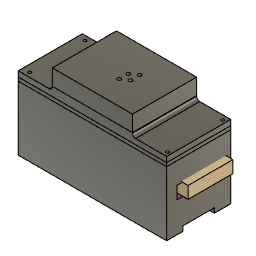
Enphase Relay Controller Unit v24 (Autodesk Fusion 360 design; units mm, degrees)
Autodesk Fusion 360 part; units mm, degrees
sketch "Device 1" plane through (0, 0, 0) normal (0, 0, 1) x (1, 0, 0)
  line L0 (0, 0) -> (58, 0)
  line L1 (58, 0) -> (58, 29)
  line L2 (58, 29) -> (0, 29)
  line L3 (0, 29) -> (0, 0)
  dimension "d1" = 58
  dimension "d2" = 29
  constraint horizontal L0
  constraint vertical L1
  constraint horizontal L2
  constraint vertical L3
  constraint coincident L0.start L3.end
  measures "d1" distance of L0.start L0.end
  measures "d2" distance of L0.start L2.end
extrude "Extrude1" add sketch "Device 1" along normal blind 1.5 makes body 1
sketch "Device 2" plane through (0, 0, 1.5) normal (0, 0, 1) x (-1, 0, 0)
  line L0 (0, -29) -> (0, 0)
  line L1 (0, 0) -> (-58, 0)
  line L2 (-58, 0) -> (-58, -29)
  line L3 (-58, -29) -> (0, -29)
  line L4 (0, -29) -> (-5, -29) construction
  line L5 (-5, -29) -> (-5, -28) construction
  line L6 (-5, -28) -> (-53, -28)
  line L7 (-53, -28) -> (-53, -25.7)
  line L8 (-53, -25.7) -> (-5, -25.7)
  line L9 (-5, -25.7) -> (-5, -28)
  line L10 (0, 0) -> (-5, 0) construction
  line L11 (-5, 0) -> (-5, -1) construction
  line L12 (-5, -1) -> (-53, -1)
  line L13 (-53, -1) -> (-53, -3.3)
  line L14 (-53, -3.3) -> (-5, -3.3)
  line L15 (-5, -3.3) -> (-5, -1)
  line L16 (-58, -29) -> (-58, -24) construction
  line L17 (-58, 0) -> (-58, -13) construction
  line L18 (-58, -24) -> (-55, -24) construction
  line L19 (-58, -13) -> (-59.5, -13) construction
  line L20 (-55, -24) -> (-59.5, -24)
  line L21 (-59.5, -24) -> (-59.5, -13)
  line L22 (-59.5, -13) -> (-55, -13)
  line L23 (-55, -13) -> (-55, -24)
  dimension "d5" = 5
  dimension "d6" = 1
  dimension "d9" = 48
  dimension "d10" = 2.3
  dimension "d11" = 5
  dimension "d12" = 1
  dimension "d13" = 48
  dimension "d14" = 2.3
  dimension "d99" = 5
  dimension "d100" = 13
  dimension "d101" = 3
  dimension "d102" = 1.5
  constraint coincident L0.start L3.end
  constraint perpendicular L0 L4
  constraint perpendicular L4 L5
  constraint horizontal L6
  constraint vertical L7
  constraint horizontal L8
  constraint vertical L9
  constraint coincident L0.end L1.start
  constraint coincident L1 L10.end
  constraint perpendicular L10 L11
  constraint horizontal L12
  constraint vertical L13
  constraint horizontal L14
  constraint vertical L15
  constraint coincident L2.end L3.start
  constraint perpendicular L3 L16
  constraint coincident L1.end L2.start
  constraint perpendicular L1 L17
  constraint perpendicular L2 L18
  constraint perpendicular L17 L19
  constraint horizontal L20
  constraint vertical L21
  constraint horizontal L22
  constraint vertical L23
  measures "d5" distance of L0.start L4.end
  measures "d6" distance of L4.end L5.end
  measures "d9" distance of L5.end L6.end
  measures "d10" distance of L5.end L8.end
  measures "d11" distance of L0.end L10.end
  measures "d12" distance of L10.end L11.end
  measures "d13" distance of L11.end L12.end
  measures "d14" distance of L11.end L14.end
  measures "d99" distance of L2.end L16.end
  measures "d100" distance of L1.end L17.end
  measures "d101" distance of L16.end L18.end
  measures "d102" distance of L17.end L19.end
extrude "Extrude2" add sketch "Device 2" along normal blind 11.12 contours L6 L7 L8 L9 | L12 L13 L14 L15 bodies 1
sketch "Device 3" plane through (0, 0, 12.62) normal (0, 0, 1) x (-1, 0, 0)
  line L0 (-5, -3.3) -> (-5, -1)
  line L1 (-5, -1) -> (-53, -1)
  line L2 (-53, -1) -> (-53, -3.3)
  line L3 (-53, -3.3) -> (-5, -3.3)
  line L4 (-5, -1) -> (-0.8, -1) construction
  line L5 (-0.8, -1) -> (-0.8, 0.45) construction
  line L6 (-0.8, 0.45) -> (-57.6, 0.45)
  line L7 (-57.6, 0.45) -> (-57.6, -31.05)
  line L8 (-57.6, -31.05) -> (-0.8, -31.05)
  line L9 (-0.8, -31.05) -> (-0.8, 0.45)
  line L10 (-57.6, 0.45) -> (-57.6, -4.72) construction
  line L11 (-57.6, -4.72) -> (-67.2, -4.72)
  line L12 (-67.2, -4.72) -> (-67.2, -29.82)
  line L13 (-67.2, -29.82) -> (-57.6, -29.82)
  line L14 (-57.6, -29.82) -> (-57.6, -4.72)
  dimension "d17" = 4.2
  dimension "d18" = 1.45
  dimension "d19" = 56.8
  dimension "d20" = 31.5
  dimension "d21" = 5.17
  dimension "d22" = 9.6
  dimension "d23" = 25.1
  constraint coincident L0.end L1.start
  constraint perpendicular L0 L4
  constraint perpendicular L4 L5
  constraint horizontal L6
  constraint vertical L7
  constraint horizontal L8
  constraint vertical L9
  constraint perpendicular L6 L10
  constraint horizontal L11
  constraint vertical L12
  constraint horizontal L13
  constraint vertical L14
  measures "d17" distance of L0.end L4.end
  measures "d18" distance of L4.end L5.end
  measures "d19" distance of L5.end L6.end
  measures "d20" distance of L5.end L8.end
  measures "d21" distance of L6.end L10.end
  measures "d22" distance of L10.end L11.end
  measures "d23" distance of L10.end L13.end
extrude "Extrude3" add sketch "Device 3" along normal blind 1.6 contours L0 L1 L2 L3 | L6 L7 L8 L9 L14 bodies 1
extrude "Extrude4" add sketch "Device 3" along normal blind 5.77 contours L7 L11 L12 L13 L14 bodies 1
sketch "Device 4" plane through (0, 0, 14.22) normal (0, 0, 1) x (-1, 0, 0)
  line L0 (-57.6, -31.05) -> (-0.8, -31.05)
  line L1 (-0.8, -31.05) -> (-0.8, 0.45)
  line L2 (-0.8, 0.45) -> (-57.6, 0.45)
  line L3 (-57.6, 0.45) -> (-57.6, -4.72)
  line L4 (-57.6, -4.72) -> (-57.6, -29.82)
  line L5 (-57.6, -29.82) -> (-57.6, -31.05)
  line L6 (-57.6, -31.05) -> (-53.8, -31.05) construction
  line L7 (-53.8, -31.05) -> (-53.8, -29.25) construction
  line L8 (-53.8, -29.25) -> (-23.9, -29.25)
  line L9 (-23.9, -29.25) -> (-23.9, -8.75)
  line L10 (-23.9, -8.75) -> (-53.8, -8.75)
  line L11 (-53.8, -8.75) -> (-53.8, -29.25)
  line L12 (-53.8, -29.25) -> (-16, -29.25) construction
  line L13 (-16, -29.25) -> (-21.5, -29.25)
  line L14 (-21.5, -29.25) -> (-21.5, -17.75)
  line L15 (-21.5, -17.75) -> (-16, -17.75)
  line L16 (-16, -17.75) -> (-16, -29.25)
  line L17 (-21.5, -29.25) -> (-8.15, -29.25) construction
  line L18 (-8.15, -29.25) -> (-14, -29.25)
  line L19 (-14, -29.25) -> (-14, -14.45)
  line L20 (-14, -14.45) -> (-8.15, -14.45)
  line L21 (-8.15, -14.45) -> (-8.15, -29.25)
  dimension "d28" = 3.8
  dimension "d29" = 1.8
  dimension "d30" = 29.9
  dimension "d31" = 20.5
  dimension "d32" = 37.8
  dimension "d33" = 5.5
  dimension "d34" = 11.5
  dimension "d35" = 13.35
  dimension "d36" = 5.85
  dimension "d37" = 14.8
  constraint coincident L0.start L5.end
  constraint perpendicular L5 L6
  constraint perpendicular L6 L7
  constraint horizontal L8
  constraint vertical L9
  constraint horizontal L10
  constraint vertical L11
  constraint perpendicular L7 L12
  constraint horizontal L13
  constraint vertical L14
  constraint horizontal L15
  constraint vertical L16
  constraint perpendicular L14 L17
  constraint horizontal L18
  constraint vertical L19
  constraint horizontal L20
  constraint vertical L21
  measures "d28" distance of L0.start L6.end
  measures "d29" distance of L6.end L7.end
  measures "d30" distance of L7.end L8.end
  measures "d31" distance of L7.end L10.end
  measures "d32" distance of L7.end L12.end
  measures "d33" distance of L12.end L13.end
  measures "d34" distance of L12.end L15.end
  measures "d35" distance of L13.end L17.end
  measures "d36" distance of L17.end L18.end
  measures "d37" distance of L17.end L20.end
extrude "Extrude5" add sketch "Device 4" along normal blind 14.6 contours L8 L9 L10 L11 bodies 1
extrude "Extrude6" add sketch "Device 4" along normal blind 10.2 contours L13 L14 L15 L16 bodies 1
extrude "Extrude7" add sketch "Device 4" along normal blind 10.2 contours L18 L19 L20 L21 bodies 1
sketch "Enclosure Base 1" plane through (0, 0, 0) normal (0, 0, 1) x (1, 0, 0)
  line L0 (0, 0) -> (83.3, 0)
  line L1 (83.3, 0) -> (83.3, 35)
  line L2 (83.3, 35) -> (0, 35)
  line L3 (0, 35) -> (0, 0)
  line L4 (83.3, 17.5) -> (83.3, 26.35) construction
  line L5 (83.3, 17.5) -> (83.3, 8.65) construction
  line L6 (83.3, 26.35) -> (0, 26.35)
  line L7 (0, 26.35) -> (0, 8.65)
  line L8 (0, 8.65) -> (83.3, 8.65)
  line L9 (83.3, 8.65) -> (83.3, 26.35)
  dimension "d44" = 83.3
  dimension "d45" = 35
  dimension "d46" = 8.85
  dimension "d47" = 8.85
  constraint horizontal L0
  constraint vertical L1
  constraint horizontal L2
  constraint vertical L3
  constraint coincident L0.start L3.end
  constraint midpoint L1 L4.start
  constraint perpendicular L2 L4
  constraint parallel L1 L5
  constraint horizontal L6
  constraint vertical L7
  constraint horizontal L8
  constraint vertical L9
  constraint coincident L3 L7.end
  measures "d44" distance of L0.start L0.end
  measures "d45" distance of L0.start L2.end
  measures "d46" distance of L4.start L4.end
  measures "d47" distance of L4.start L5.end
extrude "Extrude8" add sketch "Enclosure Base 1" along normal blind 5 separate body makes body 2
extrude "Extrude9" cut sketch "Enclosure Base 1" along normal blind 2.68 contours L1 L3 L6 L7 L8 L9 bodies 2
move_body "Move1" bodies 1 to x (1, 0, 0) y (0, 1, 0) z (0, 0, 1) at (25.3, 0, 5)
extrude "Extrude10" add 1 faces at (27.7667, 0, 1.6667) along direction (0, -1, 0) blind 0.5 on bodies 2 bodies 2
extrude "Extrude11" add 1 faces at (55.5333, 35, 1.6667) along direction (0, 1, 0) blind 0.5 on bodies 2 bodies 2
move_body "Move2" bodies 1 to x (1, 0, 0) y (0, 1, 0) z (0, 0, 1) at (-5.25, 2.12, 0)
sketch "Enclosure Base 2" plane through (0, 0, 5) normal (0, 0, 1) x (-1, 0, 0)
  line L0 (-83.3, 0.5) -> (-83.3, -35.5)
  line L1 (-83.3, -35.5) -> (0, -35.5)
  line L2 (0, -35.5) -> (0, 0.5)
  line L3 (0, 0.5) -> (-83.3, 0.5)
  line L4 (-20.05, -31.12) -> (-20.05, -35.5) construction
  line L5 (-20.05, -2.12) -> (-20.05, 0.5) construction
  line L6 (-78.05, -2.12) -> (-78.05, 0.5) construction
  line L7 (-78.05, -2.12) -> (-78.3, -2.123) construction
  line L8 (-20.05, -31.12) -> (-20.05, -31.37) construction
  line L9 (-20.05, -31.37) -> (-19.8, -31.37) construction
  line L10 (-20.05, -2.12) -> (-20.05, -1.87) construction
  line L11 (-20.05, -1.87) -> (-19.8, -1.87) construction
  line L12 (-78.05, 0.5) -> (-78.05, -35.5) construction
  line L13 (0, -4.123) -> (-5, -4.123) construction
  line L14 (-19.8, -2.123) -> (-19.8, -2.823) construction
  line L15 (-19.8, -31.37) -> (-19.8, -32.07) construction
  line L16 (-78.3, -2.123) -> (-78.3, -2.823) construction
  line L17 (-5, -4.123) -> (-5, -4.823) construction
  line L18 (-19.8, -32.07) -> (-78.3, -32.07)
  line L19 (-78.3, -32.07) -> (-78.3, -2.823)
  line L20 (-78.3, -2.823) -> (-19.8, -2.823)
  line L21 (-19.8, -32.07) -> (-19.8, -2.823)
  line L22 (-19.8, -2.823) -> (-19.8, -4.823) construction
  line L23 (-19.8, -32.07) -> (-19.8, -30.07) construction
  line L24 (-19.8, -30.07) -> (-5, -30.07)
  line L25 (-5, -30.07) -> (-5, -4.823)
  line L26 (-5, -4.823) -> (-19.8, -4.823)
  line L27 (-19.8, -4.823) -> (-19.8, -30.07)
  line L28 (-19.8, -4.823) -> (-9.8, -4.823) construction
  line L29 (-19.8, -30.07) -> (-9.8, -30.07) construction
  line L30 (-9.8, -30.07) -> (-19.8, -30.07)
  line L31 (-19.8, -30.07) -> (-19.8, -32.07)
  line L32 (-19.8, -32.07) -> (-9.8, -32.07)
  line L33 (-9.8, -32.07) -> (-9.8, -30.07)
  line L34 (-19.8, -2.823) -> (-9.8, -2.823)
  line L35 (-9.8, -2.823) -> (-9.8, -4.823)
  line L36 (-9.8, -4.823) -> (-19.8, -4.823)
  line L37 (-19.8, -4.823) -> (-19.8, -2.823)
  point P0 (-20.05, -31.12)
  point P1 (-20.05, -2.12)
  point P2 (-78.05, -2.12)
  point P3 (-78.05, -2.12)
  dimension "d69" = 0.25
  dimension "d72" = 0.25
  dimension "d73" = 0.25
  dimension "d74" = 0.25
  dimension "d75" = 0.25
  dimension "d78" = 5
  dimension "d85" = 0.7
  dimension "d87" = 0.7
  dimension "d89" = 0.7
  dimension "d90" = 0.7
  dimension "d91" = 2
  dimension "d92" = 2
  dimension "d93" = 10
  dimension "d94" = 10
  constraint coincident P0 L4.start
  constraint coincident L1 L4.end
  constraint perpendicular L1 L4
  constraint coincident P1 L5.start
  constraint coincident L3 L5.end
  constraint perpendicular L3 L5
  constraint coincident P3 P2
  constraint coincident L3 L6.end
  constraint perpendicular L3 L6
  constraint parallel L4 L8
  constraint perpendicular L8 L9
  constraint parallel L5 L10
  constraint perpendicular L10 L11
  constraint coincident L1 L12.end
  constraint perpendicular L1 L12
  constraint coincident L2 L13.start
  constraint perpendicular L2 L13
  constraint perpendicular L9 L15
  constraint horizontal L18
  constraint vertical L19
  constraint horizontal L20
  constraint perpendicular L20 L21
  constraint perpendicular L20 L22
  constraint perpendicular L9 L23
  constraint horizontal L24
  constraint vertical L25
  constraint horizontal L26
  constraint vertical L27
  constraint perpendicular L27 L28
  constraint perpendicular L21 L29
  constraint horizontal L30
  constraint vertical L31
  constraint horizontal L32
  constraint vertical L33
  constraint horizontal L34
  constraint vertical L35
  constraint horizontal L36
  constraint vertical L37
  measures "d69" distance of P3 L7.end
  measures "d72" distance of P0 L8.end
  measures "d73" distance of L8.end L9.end
  measures "d74" distance of P1 L10.end
  measures "d75" distance of L10.end L11.end
  measures "d78" distance of L13.start L13.end
  measures "d85" distance of L14.start L14.end
  measures "d87" distance of L9.end L15.end
  measures "d89" distance of L7.end L16.end
  measures "d90" distance of L13.end L17.end
  measures "d91" distance of L14.end L22.end
  measures "d92" distance of L15.end L23.end
  measures "d93" distance of L22.end L28.end
  measures "d94" distance of L23.end L29.end
extrude "Extrude16" add sketch "Enclosure Base 2" along normal blind 2.5 contours L21 L24 L30 L31 L32 L33 | L21 L26 L34 L35 L36 L37 bodies 2
extrude "Extrude17" add sketch "Enclosure Base 2" along normal blind 14 bodies 2
move_body "Move4" bodies 1 to x (1, 0, 0) y (0, 1, 0) z (0, 0, 1) at (0, 0.825, 0)
sketch "Device 5" plane through (0, 0, 6.5) normal (0, 0, 1) x (-1, 0, 0)
  line L0 (-25.05, -6.245) -> (-73.05, -6.245)
  line L1 (-73.05, -6.245) -> (-73.05, -3.945)
  line L2 (-73.05, -3.945) -> (-25.05, -3.945)
  line L3 (-25.05, -3.945) -> (-25.05, -6.245)
  line L4 (-25.05, -28.645) -> (-25.05, -30.945)
  line L5 (-25.05, -30.945) -> (-73.05, -30.945)
  line L6 (-73.05, -30.945) -> (-73.05, -28.645)
  line L7 (-73.05, -28.645) -> (-25.05, -28.645)
  line L8 (-20.05, -31.945) -> (-20.05, -2.945)
  line L9 (-20.05, -2.945) -> (-78.05, -2.945)
  line L10 (-78.05, -2.945) -> (-78.05, -31.945)
  line L11 (-78.05, -31.945) -> (-20.05, -31.945)
  line L12 (-78.05, -31.945) -> (-78.05, -26.945) construction
  line L13 (-78.05, -2.945) -> (-78.05, -15.945) construction
  line L14 (-78.05, -15.945) -> (-80.05, -15.945) construction
  line L15 (-78.05, -26.945) -> (-75.05, -26.945) construction
  line L16 (-75.05, -26.945) -> (-80.05, -26.945)
  line L17 (-80.05, -26.945) -> (-80.05, -15.945)
  line L18 (-80.05, -15.945) -> (-75.05, -15.945)
  line L19 (-75.05, -15.945) -> (-75.05, -26.945)
  dimension "d103" = 5
  dimension "d104" = 13
  dimension "d105" = 2
  dimension "d106" = 3
  constraint coincident L10.end L11.start
  constraint perpendicular L11 L12
  constraint coincident L9.end L10.start
  constraint perpendicular L9 L13
  constraint perpendicular L10 L14
  constraint perpendicular L10 L15
  constraint horizontal L16
  constraint vertical L17
  constraint horizontal L18
  constraint vertical L19
  measures "d103" distance of L10.end L12.end
  measures "d104" distance of L9.end L13.end
  measures "d105" distance of L13.end L14.end
  measures "d106" distance of L12.end L15.end
extrude "Extrude18" add sketch "Device 5" along normal blind 3 contours L10 L16 L17 L18 | L10 L16 L18 L19 bodies 1
sketch "Enclosure Base 3" plane through (78.3, 0, 0) normal (-1, 0, 0) x (0, -1, 0)
  line L0 (-32.07, 5) -> (-2.823, 5)
  line L1 (-2.823, 5) -> (-2.823, 19)
  line L2 (-2.823, 19) -> (-32.07, 19)
  line L3 (-32.07, 19) -> (-32.07, 5)
  line L4 (-32.07, 5) -> (-27.57, 5) construction
  line L5 (-2.823, 19) -> (-15.323, 19) construction
  line L6 (-27.57, 5) -> (-15.323, 5)
  line L7 (-15.323, 5) -> (-15.323, 19)
  line L8 (-15.323, 19) -> (-27.57, 19)
  line L9 (-27.57, 19) -> (-27.57, 5)
  dimension "d109" = 4.5
  dimension "d110" = 12.5
  constraint coincident L0.start L3.end
  constraint perpendicular L3 L4
  constraint coincident L1.end L2.start
  constraint perpendicular L1 L5
  constraint horizontal L6
  constraint vertical L7
  constraint horizontal L8
  constraint vertical L9
  measures "d109" distance of L0.start L4.end
  measures "d110" distance of L1.end L5.end
extrude "Extrude19" cut sketch "Enclosure Base 3" against normal blind 2 contours L0 L2 L6 L7 L8 L9 bodies 2
sketch "Device 6" plane through (0, 0, 17.62) normal (0, 0, -1) x (1, 0, 0)
  line L0 (73.05, -6.245) -> (25.05, -6.245)
  line L1 (25.05, -6.245) -> (25.05, -3.945)
  line L2 (25.05, -3.945) -> (73.05, -3.945)
  line L3 (73.05, -3.945) -> (73.05, -6.245)
  line L4 (25.05, -30.945) -> (25.05, -28.645)
  line L5 (25.05, -28.645) -> (73.05, -28.645)
  line L6 (73.05, -28.645) -> (73.05, -30.945)
  line L7 (73.05, -30.945) -> (25.05, -30.945)
  line L8 (20.85, -33.995) -> (77.65, -33.995)
  line L9 (77.65, -33.995) -> (77.65, -32.765)
  line L10 (77.65, -32.765) -> (87.25, -32.765)
  line L11 (87.25, -32.765) -> (87.25, -7.665)
  line L12 (87.25, -7.665) -> (77.65, -7.665)
  line L13 (77.65, -7.665) -> (77.65, -2.495)
  line L14 (77.65, -2.495) -> (20.85, -2.495)
  line L15 (20.85, -2.495) -> (20.85, -33.995)
  line L16 (87.25, -7.665) -> (77.65, -7.665)
  line L17 (77.65, -7.665) -> (77.65, -32.765)
  line L18 (77.65, -32.765) -> (87.25, -32.765)
  line L19 (87.25, -32.765) -> (87.25, -7.665)
  constraint horizontal L16
  constraint vertical L17
  constraint horizontal L18
  constraint vertical L19
  constraint coincident L9.end L10.start
  constraint coincident L11.end L12.start
extrude "Extrude20" add sketch "Device 6" along normal blind 1 contours L10 L11 L12 L16 L17 L18 L19 bodies 1
move_body "Move5" bodies 1 to x (1, 0, 0) y (0, 1, 0) z (0, 0, 1) at (0, 0, 1.405)
sketch "Enclosure Base 4" plane through (0, 0, 19) normal (0, 0, 1) x (-1, 0, 0)
  line L0 (0, 0.5) -> (-83.3, 0.5)
  line L1 (-83.3, 0.5) -> (-83.3, -35.5)
  line L2 (-83.3, -35.5) -> (0, -35.5)
  line L3 (0, -35.5) -> (0, 0.5)
  line L4 (-78.3, -27.57) -> (-80.3, -27.57)
  line L5 (-80.3, -27.57) -> (-80.3, -15.323)
  line L6 (-80.3, -15.323) -> (-78.3, -15.323)
  line L7 (-78.3, -15.323) -> (-78.3, -2.823)
  line L8 (-78.3, -2.823) -> (-9.8, -2.823)
  line L9 (-9.8, -2.823) -> (-9.8, -4.823)
  line L10 (-9.8, -4.823) -> (-5, -4.823)
  line L11 (-5, -4.823) -> (-5, -30.07)
  line L12 (-5, -30.07) -> (-9.8, -30.07)
  line L13 (-9.8, -30.07) -> (-9.8, -32.07)
  line L14 (-9.8, -32.07) -> (-78.3, -32.07)
  line L15 (-78.3, -2.823) -> (-78.3, -5.323) construction
  line L16 (-78.3, -15.323) -> (-78.3, -5.323)
  line L17 (-80.3, -15.323) -> (-78.3, -15.323)
  line L18 (-80.3, -27.57) -> (-80.3, -15.323)
  line L19 (-78.3, -27.57) -> (-80.3, -27.57)
  line L20 (-78.3, -5.323) -> (-83.3, -5.323)
  line L21 (-78.3, -27.57) -> (-78.3, -33.07)
  line L22 (-78.3, -33.07) -> (-83.3, -33.0453)
  line L23 (-83.3, -33.0453) -> (-83.3, -5.323)
  dimension "d116" = 2.5
  constraint coincident L7.end L8.start
  constraint perpendicular L8 L15
  constraint coincident L6.end L7.start
  constraint coincident L5.end L6.start
  constraint coincident L4.end L5.start
  constraint coincident L4.start L19.start
  constraint horizontal L20
  constraint coincident L1 L20.end
  constraint perpendicular L14 L21
  constraint coincident L1 L22.end
  measures "d116" distance of L7.end L15.end
extrude "Extrude23" cut sketch "Enclosure Base 4" against normal blind 2 contours L1 L4 L5 L6 L7 L16 L17 L18 L19 L20 L21 L22 L23 bodies 2
sketch "Enclosure Base 6" plane through (0, 0, 19) normal (0, 0, 1) x (-1, 0, 0)
  line L0 (-83.3, -5.323) -> (-78.3, -5.323)
  line L1 (-78.3, -5.323) -> (-78.3, -2.823)
  line L2 (-78.3, -2.823) -> (-9.8, -2.823)
  line L3 (-9.8, -2.823) -> (-9.8, -4.823)
  line L4 (-9.8, -4.823) -> (-5, -4.823)
  line L5 (-5, -4.823) -> (-5, -30.07)
  line L6 (-5, -30.07) -> (-9.8, -30.07)
  line L7 (-9.8, -30.07) -> (-9.8, -32.07)
  line L8 (-9.8, -32.07) -> (-78.3, -32.07)
  line L9 (-78.3, -32.07) -> (-78.3, -33.07)
  line L10 (-78.3, -33.07) -> (-83.3, -33.0453)
  line L11 (-83.3, -33.0453) -> (-83.3, -35.5)
  line L12 (-83.3, -35.5) -> (0, -35.5)
  line L13 (0, -35.5) -> (0, 0.5)
  line L14 (0, 0.5) -> (-83.3, 0.5)
  line L15 (-83.3, 0.5) -> (-83.3, -5.323)
  line L16 (0, 0.5) -> (0, -35.5)
  line L17 (-83.3, -5.323) -> (-79.3, -5.323)
  line L18 (-83.3, -33.0453) -> (-79.288, -33.0651)
  line L19 (-83.3, -35.5) -> (-83.3, -33.0453)
  line L20 (-83.3, -5.323) -> (-83.3, 0.5)
  line L21 (-9.8, -1) -> (-79.3, -1)
  line L22 (0, -35.5) -> (-83.3, -35.5)
  line L23 (-79.3, -5.323) -> (-79.3, -1)
  line L24 (-9.8, -1) -> (-9.8, -4.823)
  line L25 (-9.8, -4.823) -> (-5, -4.823)
  line L26 (-5, -4.823) -> (-5, -30.07)
  line L27 (-5, -30.07) -> (-9.8, -30.07)
  line L28 (-83.3, 0.5) -> (0, 0.5)
  line L29 (-9.8, -30.07) -> (-9.8, -34)
  line L30 (-79.288, -33.0651) -> (-79.3, -34)
  line L31 (-9.8, -34) -> (-79.3, -34)
  dimension "d125" = 4
  constraint coincident L13.end L14.start
  constraint coincident L12.end L13.start
  constraint coincident L0.start L15.end
  constraint perpendicular L1 L17
  constraint coincident L10 L18.end
  constraint coincident L10.end L11.start
  constraint coincident L11.end L12.start
  constraint coincident L14.end L15.start
  constraint vertical L23
  constraint coincident L6.end L7.start
  constraint coincident L3.end L4.start
  constraint perpendicular L4 L24
  constraint coincident L4.end L5.start
  constraint coincident L5.end L6.start
  constraint parallel L7 L29
  measures "d125" distance of L0.start L17.end
extrude "Extrude24" add sketch "Enclosure Base 6" along normal blind 5 contours L0 L3 L4 L5 L6 L7 L10 L11 L12 L13 L14 L15 L16 L17 L18 L19 L20 L21 L22 L23 L24 L25 L26 L27 L28 L29 L30 L31 bodies 2
sketch "Enclosure Base 7" plane through (0, 0, 24) normal (0, 0, 1) x (-1, 0, 0)
  line L0 (-9.8, -1) -> (-9.8, -4.823)
  line L1 (-9.8, -4.823) -> (-5, -4.823)
  line L2 (-5, -4.823) -> (-5, -30.07)
  line L3 (-5, -30.07) -> (-9.8, -30.07)
  line L4 (-9.8, -30.07) -> (-9.8, -34)
  line L5 (-9.8, -34) -> (-79.3, -34)
  line L6 (-79.3, -34) -> (-79.288, -33.0651)
  line L7 (-79.288, -33.0651) -> (-83.3, -33.0453)
  line L8 (-83.3, -33.0453) -> (-83.3, -35.5)
  line L9 (-83.3, -35.5) -> (0, -35.5)
  line L10 (0, -35.5) -> (0, 0.5)
  line L11 (0, 0.5) -> (-83.3, 0.5)
  line L12 (-83.3, 0.5) -> (-83.3, -5.323)
  line L13 (-83.3, -5.323) -> (-79.3, -5.323)
  line L14 (-79.3, -5.323) -> (-79.3, -1)
  line L15 (-79.3, -1) -> (-9.8, -1)
  line L16 (0, -35.5) -> (0, 0.5)
  line L17 (0, 0.5) -> (-83.3, 0.5)
  line L18 (-83.3, 0.5) -> (-83.3, -35.5)
  line L19 (-83.3, -35.5) -> (0, -35.5)
  line L20 (-9.8, -4.823) -> (-5, -4.823)
  line L21 (-5, -4.823) -> (-5, -30.07)
  line L22 (-5, -30.07) -> (-9.8, -30.07)
  line L23 (-9.8, -30.07) -> (-9.8, -34)
  line L24 (-79.3, -34) -> (-9.8, -34)
  line L25 (-79.3, -34) -> (-79.3, -1)
  line L26 (-79.3, -1) -> (-9.8, -1)
  line L27 (-9.8, -1) -> (-9.8, -4.823)
  constraint coincident L9.end L10.start
  constraint coincident L10.end L11.start
  constraint coincident L11.end L12.start
  constraint coincident L8.end L9.start
  constraint coincident L0.end L1.start
  constraint coincident L1.end L2.start
  constraint coincident L2.end L3.start
  constraint coincident L3.end L4.start
  constraint coincident L4.end L5.start
  constraint coincident L5.end L6.start
  constraint coincident L14.end L15.start
  constraint coincident L0.start L15.end
extrude "Extrude25" add sketch "Enclosure Base 7" along normal blind 12 contours L0 L1 L2 L3 L4 L5 L7 L8 L9 L10 L11 L12 L13 L14 L15 L16 L17 L18 L19 L20 L21 L22 L23 L24 L25 L26 L27 | L7 L13 L18 L25 bodies 2
sketch "Lid Base 1" plane through (0, 0, 36) normal (0, 0, 1) x (-1, 0, 0)
  line L0 (-9.8, -34) -> (-79.3, -34)
  line L1 (-79.3, -34) -> (-79.3, -1)
  line L2 (-79.3, -1) -> (-9.8, -1)
  line L3 (-9.8, -4.823) -> (-5, -4.823)
  line L4 (-5, -4.823) -> (-5, -30.07)
  line L5 (-5, -30.07) -> (-9.8, -30.07)
  line L6 (-9.8, -30.07) -> (-9.8, -34)
  line L7 (-83.3, -35.5) -> (0, -35.5)
  line L8 (0, -35.5) -> (0, 0.5)
  line L9 (0, 0.5) -> (-83.3, 0.5)
  line L10 (-83.3, 0.5) -> (-83.3, -35.5)
  line L11 (0, -2) -> (-4, -2) construction
  line L12 (0, -35.5) -> (0, -33) construction
  line L13 (0, -33) -> (-4, -33) construction
  line L14 (-83.3, -35.5) -> (-81.3, -35.5) construction
  line L15 (-83.3, 0.5) -> (-81.3, 0.5) construction
  line L16 (-81.3, 0.5) -> (-81.3, -2) construction
  line L17 (-81.3, -35.5) -> (-81.3, -33) construction
  line L18 (0, 0.5) -> (0, -2) construction
  circle A0 centre (-4, -33) radius 0.8
  circle A1 centre (-4, -2) radius 0.8
  circle A2 centre (-81.3, -33) radius 0.8
  circle A3 centre (-81.3, -2) radius 0.8
  line L19 (0, 0.5) -> (-83.3, 0.5)
  line L20 (-83.3, 0.5) -> (-83.3, -35.5)
  line L21 (-83.3, -35.5) -> (0, -35.5)
  line L22 (0, -35.5) -> (0, 0.5)
  line L23 (-9.8, -34) -> (-9.9, -34) construction
  line L24 (-9.9, -34) -> (-9.9, -33.9) construction
  line L25 (-9.8, -1) -> (-9.9, -1) construction
  line L26 (-9.9, -1) -> (-9.9, -1.1) construction
  line L27 (-79.3, -1) -> (-79.3, -1.1) construction
  line L28 (-79.3, -1.1) -> (-79.2, -1.1) construction
  line L29 (-79.2, -1.1) -> (-79.2, -4.1)
  line L30 (-9.9, -1.1) -> (-9.9, -4.1)
  line L31 (-79.2, -1.1) -> (-9.9, -1.1)
  line L32 (-9.9, -4.1) -> (-79.2, -4.1)
  line L33 (-79.3, -34) -> (-79.2, -34) construction
  line L34 (-79.2, -34) -> (-79.2, -33.9) construction
  line L35 (-79.2, -33.9) -> (-79.2, -30.9)
  line L36 (-9.9, -33.9) -> (-9.9, -30.9)
  line L37 (-9.9, -30.9) -> (-79.2, -30.9)
  line L38 (0, 0.5) -> (0, -9.5) construction
  line L39 (0, -9.5) -> (-10, -9.5) construction
  line L40 (0, -35.5) -> (0, -25.5) construction
  line L41 (0, -25.5) -> (-10, -25.5) construction
  line L42 (-10, -25.5) -> (-45, -25.5)
  line L43 (-45, -25.5) -> (-45, -9.5)
  line L44 (-45, -9.5) -> (-10, -9.5)
  line L45 (-10, -9.5) -> (-10, -25.5)
  line L46 (-79.2, -33.9) -> (-9.9, -33.9)
  line L47 (-10, -25.5) -> (-28, -25.5) construction
  line L48 (-28, -25.5) -> (-28, -9.5)
  line L49 (0, -35.5) -> (-25, -35.5) construction
  line L50 (-25, -35.5) -> (-25, -29) construction
  circle A4 centre (-25, -29) radius 0.8
  line L51 (0, 0.5) -> (-25, 0.5) construction
  line L52 (-25, 0.5) -> (-25, -6) construction
  circle A5 centre (-25, -6) radius 0.8
  line L53 (-83.3, -35.5) -> (-58.3, -35.5) construction
  line L54 (-83.3, 0.5) -> (-58.3, 0.5) construction
  line L55 (-58.3, -35.5) -> (-58.3, -29) construction
  line L56 (-58.3, 0.5) -> (-58.3, -6) construction
  circle A6 centre (-58.3, -29) radius 0.8
  circle A7 centre (-58.3, -6) radius 0.8
  dimension "d135" = 4
  dimension "d136" = 2.5
  dimension "d137" = 4
  dimension "d140" = 2
  dimension "d142" = 2
  dimension "d143" = 2.5
  dimension "d144" = 2.5
  dimension "d145" = 2.5
  dimension "d149" = 1.6
  dimension "d150" = 1.6
  dimension "d151" = 1.6
  dimension "d152" = 1.6
  dimension "d155" = 0.1
  dimension "d156" = 0.1
  dimension "d157" = 0.1
  dimension "d158" = 0.1
  dimension "d160" = 0.1
  dimension "d161" = 0.1
  dimension "d162" = 3
  dimension "d163" = 3
  dimension "d164" = 0.1
  dimension "d165" = 0.1
  dimension "d166" = 3
  dimension "d167" = 3
  dimension "d168" = 10
  dimension "d169" = 10
  dimension "d170" = 10
  dimension "d171" = 10
  dimension "d172" = 35
  dimension "d179" = 18
  dimension "d180" = 25
  dimension "d181" = 6.5
  dimension "d182" = 1.6
  dimension "d183" = 25
  dimension "d184" = 6.5
  dimension "d185" = 1.6
  dimension "d186" = 25
  dimension "d187" = 25
  dimension "d188" = 6.5
  dimension "d189" = 6.5
  dimension "d190" = 1.6
  dimension "d191" = 1.6
  constraint coincident L8 L11.start
  constraint coincident L7.end L8.start
  constraint perpendicular L7 L12
  constraint perpendicular L8 L13
  constraint coincident L7.start L10.end
  constraint perpendicular L10 L14
  constraint coincident L9.end L10.start
  constraint perpendicular L10 L15
  constraint perpendicular L15 L16
  constraint perpendicular L14 L17
  constraint coincident L8.end L9.start
  constraint perpendicular L11 L18
  constraint coincident L13.end A0.centre
  constraint coincident L11.end A1.centre
  constraint coincident L17.end A2.centre
  constraint coincident L16.end A3.centre
  constraint horizontal L19
  constraint vertical L20
  constraint horizontal L21
  constraint vertical L22
  constraint coincident L0.start L6.end
  constraint coincident L0.end L1.start
  constraint coincident L1.end L2.start
  constraint coincident L2.end L25.start
  constraint perpendicular L23 L24
  constraint horizontal L25
  constraint perpendicular L25 L26
  constraint perpendicular L27 L28
  constraint perpendicular L28 L29
  constraint perpendicular L30 L31
  constraint perpendicular L29 L32
  constraint perpendicular L1 L33
  constraint perpendicular L0 L34
  constraint parallel L1 L35
  constraint parallel L6 L36
  constraint perpendicular L19 L38
  constraint perpendicular L38 L39
  constraint parallel L22 L40
  constraint perpendicular L22 L41
  constraint horizontal L42
  constraint vertical L43
  constraint horizontal L44
  constraint vertical L45
  constraint perpendicular L45 L47
  constraint coincident L44 L48.end
  constraint perpendicular L44 L48
  constraint perpendicular L22 L49
  constraint perpendicular L46 L50
  constraint coincident L50.end A4.centre
  constraint perpendicular L22 L51
  constraint perpendicular L31 L52
  constraint coincident L52.end A5.centre
  constraint perpendicular L20 L53
  constraint perpendicular L16 L54
  constraint perpendicular L53 L55
  constraint perpendicular L32 L56
  constraint coincident L55.end A6.centre
  constraint coincident L56.end A7.centre
  measures "d135" distance of L11.start L11.end
  measures "d136" distance of L7.end L12.end
  measures "d137" distance of L12.end L13.end
  measures "d140" distance of L7.start L14.end
  measures "d142" distance of L9.end L15.end
  measures "d143" distance of L15.end L16.end
  measures "d144" distance of L14.end L17.end
  measures "d145" distance of L8.end L11.start
  measures "d149" diameter of A0
  measures "d150" diameter of A1
  measures "d151" diameter of A2
  measures "d152" diameter of A3
  measures "d155" distance of L0.start L23.end
  measures "d156" distance of L23.end L24.end
  measures "d157" distance of L2.end L25.end
  measures "d158" distance of L25.end L26.end
  measures "d160" distance of L1.end L27.end
  measures "d161" distance of L27.end L28.end
  measures "d162" distance of L28.end L29.end
  measures "d163" distance of L26.end L30.end
  measures "d164" distance of L0.end L33.end
  measures "d165" distance of L33.end L34.end
  measures "d166" distance of L34.end L35.end
  measures "d167" distance of L24.end L36.end
  measures "d168" distance of L8.end L38.end
  measures "d169" distance of L38.end L39.end
  measures "d170" distance of L7.end L40.end
  measures "d171" distance of L40.end L41.end
  measures "d172" distance of L41.end L42.end
  measures "d179" distance of L41.end L47.end
  measures "d180" distance of L7.end L49.end
  measures "d181" distance of L49.end L50.end
  measures "d182" diameter of A4
  measures "d183" distance of L8.end L51.end
  measures "d184" distance of L51.end L52.end
  measures "d185" diameter of A5
  measures "d186" distance of L7.start L53.end
  measures "d187" distance of L9.end L54.end
  measures "d188" distance of L53.end L55.end
  measures "d189" distance of L54.end L56.end
  measures "d190" diameter of A6
  measures "d191" diameter of A7
extrude "Extrude26" cut sketch "Lid Base 1" against normal blind 8 contours A0 | A1 | A2 | A3 bodies 2
extrude "Extrude27" add sketch "Lid Base 1" against normal blind 2 separate body contours L29 L30 L31 L32 | L35 L36 L37 L46 makes body 3 at (56.1, 31.9, 36) makes body 4 at (56.1, 2.1, 36)
extrude "Extrude28" add sketch "Lid Base 1" along normal blind 2 contours L7 L8 L9 L10 L19 L20 L21 L22 | L29 L30 L31 L32 | L35 L36 L37 L46 | A4 | A5 | A6 | A7 bodies 3 4
sketch "Lid 1" plane through (0, 0, 38) normal (0, 0, 1) x (-1, 0, 0)
  line L0 (0, -35.5) -> (0, 0.5)
  line L1 (0, 0.5) -> (-83.3, 0.5)
  line L2 (-83.3, 0.5) -> (-83.3, -35.5)
  line L3 (-83.3, -35.5) -> (0, -35.5)
  circle A0 centre (-4, -33) radius 0.8
  circle A1 centre (-81.3, -33) radius 0.8
  circle A2 centre (-4, -2) radius 0.8
  circle A3 centre (-81.3, -2) radius 0.8
  circle A4 centre (-25, -29) radius 0.8
  circle A5 centre (-25, -6) radius 0.8
  circle A6 centre (-58.3, -29) radius 0.8
  circle A7 centre (-58.3, -6) radius 0.8
  line L4 (0, -35.5) -> (-83.3, -35.5)
  line L5 (-83.3, -35.5) -> (-83.3, 0.5)
  line L6 (-83.3, 0.5) -> (0, 0.5)
  line L7 (0, 0.5) -> (0, -35.5)
  line L8 (-28, -25.5) -> (-55, -25.5)
  line L9 (-55, -25.5) -> (-55, -9.5)
  line L10 (-55, -9.5) -> (-28, -9.5)
  line L11 (-28, -9.5) -> (-28, -25.5)
  point P0 (-25, -29)
  point P1 (-25, -6)
  point P2 (-58.3, -29)
  point P3 (-58.3, -6)
  point P4 (0, -35.5)
  point P5 (-83.3, 0.5)
  point P6 (-28, -25.5)
  dimension "d192" = 27
  dimension "d193" = 16
  constraint coincident P0 A4.centre
  constraint coincident P1 A5.centre
  constraint coincident P2 A6.centre
  constraint coincident P3 A7.centre
  constraint horizontal L4
  constraint vertical L5
  constraint horizontal L6
  constraint vertical L7
  constraint coincident P5 L1.end
  constraint coincident P4 L0.start
  constraint horizontal L8
  constraint vertical L9
  constraint horizontal L10
  constraint vertical L11
  constraint coincident P6 L8.start
  measures "d192" distance of P6 L8.end
  measures "d193" distance of P6 L10.end
extrude "Extrude29" add sketch "Lid 1" along normal blind 3 separate body makes body 5
sketch "Lid " plane through (0, 0, 41) normal (0, 0, 1) x (-1, 0, 0)
  circle A0 centre (-25, -29) radius 0.8
  circle A1 centre (-4, -2) radius 0.8
  circle A2 centre (-4, -33) radius 0.8
  circle A3 centre (-25, -6) radius 0.8
  circle A4 centre (-58.3, -29) radius 0.8
  circle A5 centre (-81.3, -2) radius 0.8
  line L0 (-55, -9.5) -> (-28, -9.5)
  line L1 (-28, -9.5) -> (-28, -25.5)
  line L2 (-28, -25.5) -> (-55, -25.5)
  line L3 (-55, -25.5) -> (-55, -9.5)
  circle A6 centre (-81.3, -33) radius 0.8
  circle A7 centre (-58.3, -6) radius 0.8
  line L4 (0, -35.5) -> (0, 0.5)
  line L5 (0, 0.5) -> (-83.3, 0.5)
  line L6 (-83.3, 0.5) -> (-83.3, -35.5)
  line L7 (-83.3, -35.5) -> (0, -35.5)
  line L8 (-64.15, -35.5) -> (-64.15, 0.5)
  line L9 (-64.15, 0.5) -> (-19.15, 0.5)
  line L10 (-19.15, 0.5) -> (-19.15, -35.5)
  line L11 (-64.15, -35.5) -> (-19.15, -35.5)
  circle A8 centre (-25, -29) radius 0.8
  circle A9 centre (-58.3, -29) radius 0.8
  circle A10 centre (-25, -6) radius 0.8
  circle A11 centre (-58.3, -6) radius 0.8
  point P0 (-25.8, -29)
  point P1 (-59.1, -29)
  point P2 (-25.8, -6)
  point P3 (-59.1, -6)
  dimension "d198" = 45
  constraint vertical L8
  constraint horizontal L9
  constraint vertical L10
  constraint coincident L5 L8.end
  constraint perpendicular L10 L11
  constraint concentric A0 A8
  constraint coincident A8 P0
  constraint concentric A4 A9
  constraint coincident A9 P1
  constraint concentric A3 A10
  constraint coincident A10 P2
  constraint concentric A7 A11
  constraint coincident A11 P3
  measures "d198" distance of L10.end L8.start
extrude "Extrude30" add sketch "Lid " along normal blind 2 contours L5 L7 L8 L9 L10 L11 bodies 3 5
fillet "Fillet2" radius 1.75 2 edges at (64.15, 17.5, 41) (19.15, 17.5, 41) on bodies 5
sketch "Lid 3" plane through (0, 0, 43) normal (0, 0, 1) x (-1, 0, 0)
  line L0 (-28, -25.5) -> (-55, -25.5)
  line L1 (-55, -25.5) -> (-55, -9.5)
  line L2 (-55, -9.5) -> (-28, -9.5)
  line L3 (-28, -9.5) -> (-28, -25.5)
  circle A0 centre (-58.3, -6) radius 0.8
  circle A1 centre (-25, -29) radius 0.8
  circle A2 centre (-58.3, -29) radius 0.8
  circle A3 centre (-25, -6) radius 0.8
  line L4 (-64.15, 0.5) -> (-64.15, -35.5)
  line L5 (-64.15, -35.5) -> (-19.15, -35.5)
  line L6 (-19.15, -35.5) -> (-19.15, 0.5)
  line L7 (-19.15, 0.5) -> (-64.15, 0.5)
  line L8 (-28, -25.5) -> (-28, -26.5) construction
  line L9 (-28, -26.5) -> (-27, -26.5) construction
  line L10 (-55, -9.5) -> (-56, -9.5) construction
  line L11 (-56, -9.5) -> (-56, -8.5) construction
  line L12 (-27, -26.5) -> (-56, -26.5)
  line L13 (-56, -26.5) -> (-56, -8.5)
  line L14 (-56, -8.5) -> (-27, -8.5)
  line L15 (-27, -8.5) -> (-27, -26.5)
  dimension "d203" = 1
  dimension "d204" = 1
  dimension "d205" = 1
  dimension "d206" = 1
  constraint coincident L0.start L3.end
  constraint perpendicular L0 L8
  constraint perpendicular L8 L9
  constraint coincident L1.end L2.start
  constraint perpendicular L1 L10
  constraint perpendicular L10 L11
  constraint horizontal L12
  constraint vertical L13
  constraint horizontal L14
  constraint vertical L15
  measures "d203" distance of L0.start L8.end
  measures "d204" distance of L8.end L9.end
  measures "d205" distance of L1.end L10.end
  measures "d206" distance of L10.end L11.end
extrude "Extrude31" add sketch "Lid 3" along normal blind 1 contours L12 L13 L14 L15 bodies 5 3
fillet "Fillet3" radius 2 4 edges at (55, 25.5, 41) (28, 25.5, 41) (55, 9.5, 41) (28, 9.5, 41) on bodies 5
fillet "Fillet4" radius 2 4 edges at (56, 26.5, 43.5) (56, 8.5, 43.5) (27, 8.5, 43.5) (27, 26.5, 43.5) on bodies 5
sketch "Lid Top 1" plane through (0, 0, 43) normal (0, 0, 1) x (-1, 0, 0)
  line L0 (-27, -10.5) -> (-27, -24.5)
  arc A0 (-29, -26.5) -> (-27, -24.5) centre (-29, -24.5) ccw
  line L1 (-29, -26.5) -> (-54, -26.5)
  arc A1 (-56, -24.5) -> (-54, -26.5) centre (-54, -24.5) ccw
  line L2 (-56, -24.5) -> (-56, -10.5)
  arc A2 (-54, -8.5) -> (-56, -10.5) centre (-54, -10.5) ccw
  line L3 (-54, -8.5) -> (-29, -8.5)
  arc A3 (-27, -10.5) -> (-29, -8.5) centre (-29, -10.5) ccw
  circle A4 centre (-25, -29) radius 0.8
  circle A5 centre (-58.3, -29) radius 0.8
  circle A6 centre (-58.3, -6) radius 0.8
  circle A7 centre (-25, -6) radius 0.8
  line L4 (-64.15, 0.5) -> (-64.15, -35.5)
  line L5 (-64.15, -35.5) -> (-19.15, -35.5)
  line L6 (-19.15, -35.5) -> (-19.15, 0.5)
  line L7 (-19.15, 0.5) -> (-64.15, 0.5)
  circle A8 centre (-25, -29) radius 0.8
  circle A9 centre (-58.3, -29) radius 0.8
  circle A10 centre (-58.3, -6) radius 0.8
  circle A11 centre (-25, -6) radius 0.8
  line L8 (-19.15, -35.5) -> (-64.15, -35.5)
  line L9 (-64.15, -35.5) -> (-64.15, 0.5)
  line L10 (-64.15, 0.5) -> (-19.15, 0.5)
  line L11 (-19.15, 0.5) -> (-19.15, -35.5)
  line L12 (-27, -26.5) -> (-27, -26.75) construction
  line L13 (-27, -26.75) -> (-26.75, -26.75) construction
  line L14 (-56, -8.5) -> (-27, -8.5) construction
  line L15 (-56, -8.5) -> (-56, -8.25) construction
  line L16 (-56, -8.25) -> (-56.25, -8.25) construction
  line L17 (-56.25, -8.25) -> (-26.75, -8.25)
  line L18 (-26.75, -8.25) -> (-26.75, -26.75)
  line L19 (-26.75, -26.75) -> (-56.25, -26.75)
  line L20 (-56.25, -26.75) -> (-56.25, -8.25)
  point P0 (-25.8, -29)
  point P1 (-59.1, -29)
  point P2 (-25.8, -6)
  point P3 (-27, -26.5)
  point P4 (-56, -8.5)
  dimension "d213" = 0.25
  dimension "d214" = 0.25
  dimension "d215" = 0.25
  dimension "d216" = 0.25
  constraint concentric A4 A8
  constraint coincident A8 P0
  constraint concentric A5 A9
  constraint coincident A9 P1
  constraint concentric A6 A10
  constraint concentric A7 A11
  constraint coincident A11 P2
  constraint horizontal L8
  constraint vertical L9
  constraint horizontal L10
  constraint vertical L11
  constraint coincident L4.start L7.end
  constraint coincident L5.end L6.start
  constraint coincident P3 L12.start
  constraint perpendicular L1 L12
  constraint perpendicular L12 L13
  constraint coincident P4 L14.start
  constraint perpendicular L14 L15
  constraint perpendicular L15 L16
  constraint horizontal L17
  constraint vertical L18
  constraint horizontal L19
  constraint vertical L20
  measures "d213" distance of P3 L12.end
  measures "d214" distance of L12.end L13.end
  measures "d215" distance of P4 L15.end
  measures "d216" distance of L15.end L16.end
extrude "Extrude32" add sketch "Lid Top 1" along normal blind 5 separate body contours L4 L5 L6 L7 L8 L9 L10 L11 makes body 6
sketch "Lid Top 2" plane through (0, 0, 48) normal (0, 0, 1) x (-1, 0, 0)
  circle A0 centre (-58.3, -29) radius 0.8
  circle A1 centre (-58.3, -6) radius 0.8
  circle A2 centre (-25, -29) radius 0.8
  circle A3 centre (-25, -6) radius 0.8
  line L0 (-26.75, -26.75) -> (-56.25, -26.75)
  line L1 (-56.25, -26.75) -> (-56.25, -8.25)
  line L2 (-56.25, -8.25) -> (-26.75, -8.25)
  line L3 (-26.75, -8.25) -> (-26.75, -26.75)
  line L4 (-19.15, 0.5) -> (-64.15, 0.5)
  line L5 (-64.15, 0.5) -> (-64.15, -35.5)
  line L6 (-64.15, -35.5) -> (-19.15, -35.5)
  line L7 (-19.15, -35.5) -> (-19.15, 0.5)
  line L8 (-19.15, -35.5) -> (-64.15, -35.5)
  line L9 (-64.15, -35.5) -> (-64.15, 0.5)
  line L10 (-64.15, 0.5) -> (-19.15, 0.5)
  line L11 (-19.15, 0.5) -> (-19.15, -35.5)
  line L12 (-64.15, -35.5) -> (-47.15, -35.5) construction
  line L13 (-47.15, -35.5) -> (-47.15, -20.5) construction
  line L14 (-47.15, -20.5) -> (-47.15, -15.42) construction
  line L15 (-47.15, -15.42) -> (-43.34, -15.42) construction
  line L16 (-43.34, -15.42) -> (-43.34, -12.88) construction
  line L17 (-43.34, -15.42) -> (-43.34, -17.96) construction
  circle A4 centre (-47.15, -20.5) radius 1
  circle A5 centre (-47.15, -15.42) radius 1
  circle A6 centre (-43.34, -17.96) radius 1
  circle A7 centre (-43.34, -12.88) radius 1
  point P0 (-19.15, -35.5)
  dimension "d219" = 17
  dimension "d220" = 15
  dimension "d221" = 5.08
  dimension "d222" = 3.81
  dimension "d223" = 2.54
  dimension "d224" = 2.54
  dimension "d225" = 2
  dimension "d226" = 2
  dimension "d227" = 2
  dimension "d228" = 2
  constraint horizontal L8
  constraint vertical L9
  constraint horizontal L10
  constraint vertical L11
  constraint coincident L4.end L5.start
  constraint coincident P0 L6.end
  constraint perpendicular L9 L12
  constraint perpendicular L0 L13
  constraint parallel L13 L14
  constraint perpendicular L14 L15
  constraint perpendicular L15 L16
  constraint perpendicular L15 L17
  constraint coincident L13.end L14.start
  constraint coincident L14.end L15.start
  constraint coincident L17.end A6.centre
  constraint coincident L16.end A7.centre
  measures "d219" distance of L5.end L12.end
  measures "d220" distance of L12.end L13.end
  measures "d221" distance of L13.end L14.end
  measures "d222" distance of L14.end L15.end
  measures "d223" distance of L15.end L16.end
  measures "d224" distance of L15.end L17.end
  measures "d225" diameter of A4
  measures "d226" diameter of A5
  measures "d227" diameter of A6
  measures "d228" diameter of A7
extrude "Extrude33" add sketch "Lid Top 2" along normal blind 4 contours A0 | A1 | A2 | A3 | L0 L1 L2 L3 | L4 L5 L6 L7 L8 L9 L10 L11 bodies 6
equation "d222 = ( 2.54 * 1.5 ) * 1 mm"
named bodies: "Device", "Enclosure Base", "Lid Base", "Lid", "Lid Top"
